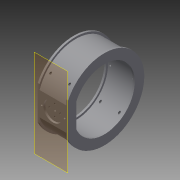
# Autodesk Inventor part: Rotorneu
Saved by Autodesk Inventor 2013 (Build 170138000, 138)
## iProperties
Created: 2013-02-04
Part Number: Rotorneu
Material: Allgemein
Document SubType Name: Modeling
Designer: Lukas
Density: 1 g/cm^3
Author: Lukas
Autodesk Inventor part; units mm, degrees
ref_plane "YZ Plane" through (0, 0, 0) normal (1, 0, 0) x (0, 1, 0)
ref_plane "XZ Plane" through (0, 0, 0) normal (0, 1, 0) x (-1, 0, 0)
ref_plane "XY Plane" through (0, 0, 0) normal (0, 0, 1) x (1, 0, 0)
sketch "Skizze1" plane through (0, 0, 0) normal (1, 0, 0) x (0, 1, 0)
  circle A0 centre (0, 0) radius 100
  circle A1 centre (0, 0) radius 85
  dimension "d9" = 200
  dimension "d10" = 170
  constraints: 2 centre point, 2 coincident
  measures "d9" diameter of A0
  measures "d10" diameter of A1
extrude "Extrusion1" add sketch "Skizze1" along normal blind 80
sketch "Skizze4" plane through (80, 0, 0) normal (1, 0, 0) x (0, 0, -1)
  circle A0 centre (0, 0) radius 85 projected
  circle A1 centre (0, 0) radius 100 projected
  line L0 (-31.225, -95) -> (31.225, -95)
  line L1 (31.225, -95) -> (31.225, -110)
  line L2 (31.225, -110) -> (-31.225, -110)
  line L3 (-31.225, -110) -> (-31.225, -95)
  dimension "d16" = 31.225
  dimension "d17" = 31.225
  dimension "d18" = 15
  constraints: 8 end point, 2 perpendicular, 1 horizontal, 1 parallel, 2 other
  measures "d16" horizontal distance of A0.centre L0.start
  measures "d17" horizontal distance of A0.centre L0.end
  measures "d18" distance of L0.end L1.end
extrude "Extrusion4" cut sketch "Skizze4" against normal blind 80 contours L0 A1 | A1 L1 L2 L3 picked at (-6.3129, -96.0634)
sketch "Skizze6" plane through (80, 0, 0) normal (1, 0, 0) x (0, 0, -1)
  circle A0 centre (0, 0) radius 85 projected
  line L0 (-31.225, -79.0569) -> (31.225, -79.0569)
  arc A1 (-31.225, -79.0569) -> (31.225, -79.0569) centre (0, 0) ccw
  constraints: 4 point on circle, 2 end point, 1 centre point, 1 coincident
extrude "Extrusion5" add sketch "Skizze6" against normal blind 80 contours L0 A0 picked at (-6.3406, -80.3194)
sketch "Skizze7" plane through (80, 0, 0) normal (1, 0, 0) x (0, 0, -1)
  arc A0 (31.225, -95) -> (-31.225, -95) centre (0, 0) ccw projected
  arc A1 (31.225, -79.0569) -> (-31.225, -79.0569) centre (0, 0) ccw projected
  line L0 (31.225, -79.0569) -> (-31.225, -79.0569) projected
  line L1 (31.225, -95) -> (44.7214, -95)
  line L2 (-31.225, -95) -> (-44.7214, -95)
  arc A2 (44.7214, -95) -> (-44.7214, -95) centre (0, 0) ccw
  line L3 (-31.225, -95) -> (31.225, -95) projected
  line L4 (-31.225, -73.6546) -> (31.225, -73.6546)
  arc A3 (31.225, -73.6546) -> (-31.225, -73.6546) centre (0, 0) ccw
  constraints: 6 end point, 4 point on circle, 3 parallel, 2 centre point, 2 coincident
extrude "Extrusion6" add sketch "Skizze7" against normal blind 5 contours A0 L2 A2 L1 | L0 A1
sketch "Skizze8" plane through (0, 0, 0) normal (-1, 0, 0) x (0, 0, 1)
  arc A0 (31.225, -95) -> (-31.225, -95) centre (0, 0) ccw projected
  arc A1 (31.225, -79.0569) -> (-31.225, -79.0569) centre (0, 0) ccw projected
  line L0 (31.225, -79.0569) -> (-31.225, -79.0569) projected
  line L1 (-31.225, -95) -> (-44.7214, -95)
  line L2 (31.225, -95) -> (44.7214, -95)
  arc A2 (44.7214, -95) -> (-44.7214, -95) centre (0, 0) ccw
  line L3 (-31.225, -95) -> (31.225, -95) projected
  line L4 (-31.225, -73.6546) -> (31.225, -73.6546)
  arc A3 (31.225, -73.6546) -> (-31.225, -73.6546) centre (0, 0) ccw
  dimension "d31" = 13.4964
  constraints: 6 end point, 4 point on circle, 3 parallel, 2 centre point, 2 coincident
  measures "d31" distance of L1.start L1.end
extrude "Extrusion7" add sketch "Skizze8" against normal blind 5 contours A0 L1 A2 L2 | L0 A1
sketch "Skizze9" plane through (80, -95, -31.225) normal (0, -1, 0) x (1, 0, 0)
  line L0 (-80, 0) -> (-80, 62.45) projected
  line L1 (-5, 0) -> (-75, 0) projected
  circle A0 centre (-40, 31.225) radius 25
  point P0 (-80, 31.225)
  dimension "d32" = 31.225
  dimension "d33" = 40
  dimension "d34" = 50
  constraints: 1 centre point, 1 coincident
  measures "d32" distance from line of L1 point (-40, 31.225)
  measures "d33" distance from line of L0 point (-40, 31.225)
  measures "d34" diameter of A0
extrude "Extrusion8" cut sketch "Skizze9" against normal blind 5
sketch "Skizze10" plane through (40, -90, 0) normal (0, -1, 0) x (1, 0, 0)
  circle A0 centre (0, 0) radius 25 projected
  point P0 (-40, 0)
  point P1 (0, 15)
  point P2 (14.3095, 0)
  point P3 (0, -14.4669)
  point P4 (-14.1949, 0)
  dimension "d37" = 15
  constraints: 1 coincident
  measures "d37" distance of point (0, 0) point (0, 15)
hole "Bohrung1" at (40, -90, 0) at (40, -90, 15) at (54.3095, -90, 0) at (40, -90, -14.4669) at (25.8051, -90, 0) direction (0, 1, 0) diameter 5 end up to face face through (28.3333, -79.0569, 10.4083) facing (0, 1, -0.0000001)
thread "Gewinde1" size "M5x0.8" class "6H" standard "ANSI Metric M Profile" full length
thread "Gewinde2" size "M5x0.8" class "6H" standard "ANSI Metric M Profile" full length
thread "Gewinde3" size "M5x0.8" class "6H" standard "ANSI Metric M Profile" full length
thread "Gewinde4" size "M5x0.8" class "6H" standard "ANSI Metric M Profile" full length
sketch "Skizze11" plane through (80, -95, -31.225) normal (0, -1, 0) x (1, 0, 0)
  line L0 (0, 62.45) -> (0, 0) projected
  line L1 (-80, 0) -> (-80, 62.45) projected
  point P0 (-80, 31.225)
  point P1 (-70, 31.225)
  point P2 (-10, 31.225)
  dimension "d54" = 10
  dimension "d55" = 10
  measures "d54" distance from line of L1 point (-70, 31.225)
  measures "d55" distance from line of L0 point (-10, 31.225)
hole "Bohrung2" at (10, -95, 0) at (70, -95, 0) direction (0, 1, 0) diameter 5 end through all
ref_plane "Arbeitsebene1" through (0, -100, 0) normal (0, -1, 0) x (1, 0, 0)
sketch "Skizze12" plane through (0, -100, 0) normal (0, -1, 0) x (1, 0, 0)
  line L0 (80, -105) -> (80, 105) projected
  line L1 (0, 105) -> (0, -105) projected
  line L2 (75, -31.225) -> (5, -31.225) projected
  line L3 (0, 0) -> (80, 0)
  point P0 (65, 65)
  point P1 (15, 65)
  point P2 (15, -65)
  point P3 (65, -65)
  point P4 (80, -44.7214)
  point P5 (80, 44.7214)
  point P6 (0, 44.7214)
  point P7 (0, -44.7214)
  dimension "d63" = 15
  dimension "d64" = 15
  dimension "d65" = 15
  dimension "d66" = 15
  dimension "d76" = 65
  dimension "d77" = 65
  dimension "d78" = 65
  dimension "d79" = 65
  constraints: 2 end point, 1 midpoint
  measures "d63" distance from line of L0 point (65, 65)
  measures "d64" distance from line of L1 point (15, 65)
  measures "d65" distance from line of L1 point (15, -65)
  measures "d66" distance from line of point (65, -65) L0
  measures "d76" distance from line of L3 point (15, -65)
  measures "d77" distance from line of L3 point (15, 65)
  measures "d78" distance from line of L3 point (65, -65)
  measures "d79" distance from line of point (65, 65) L3
hole "Bohrung3" at (65, -100, 65) at (15, -100, 65) at (15, -100, -65) at (65, -100, -65) direction (0, 1, 0) diameter 5 end through all
thread "Gewinde5" size "M5x0.8" class "6H" standard "ANSI Metric M Profile" full length
thread "Gewinde6" size "M5x0.8" class "6H" standard "ANSI Metric M Profile" full length
thread "Gewinde7" size "M5x0.8" class "6H" standard "ANSI Metric M Profile" full length
thread "Gewinde8" size "M5x0.8" class "6H" standard "ANSI Metric M Profile" full length
thread "Gewinde9" size "M5x0.8" class "6H" standard "ANSI Metric M Profile" full length
thread "Gewinde10" size "M5x0.8" class "6H" standard "ANSI Metric M Profile" full length
thread "Gewinde11" size "M5x0.8" class "6H" standard "ANSI Metric M Profile" full length
thread "Gewinde12" size "M5x0.8" class "6H" standard "ANSI Metric M Profile" full length
